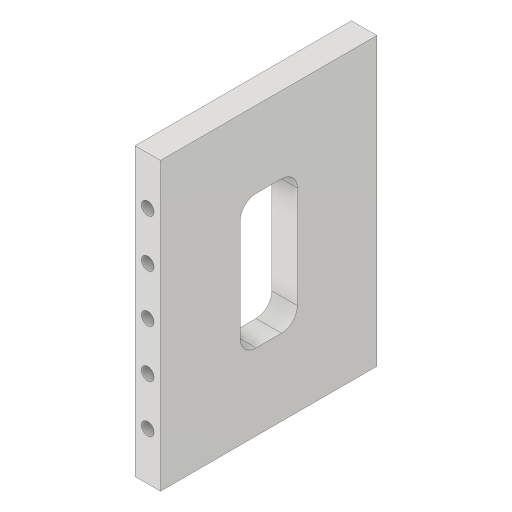
# Autodesk Inventor part: Box_Side
Saved by Autodesk Inventor 2023.2 (Build 272271000, 271)
## iProperties
Created: 2021-07-28
Part Number: Box_Side
Material: LCP 플라스틱
Document SubType Name: Modeling
Designer: user
Density: 1.626 g/cm^3
Appearance: 매끄러움 - 흰색
Mass: 8.3481 g
Surface Area: 40.5022 cm^2
Volume: 5.13413 cm^3
Author: user
Autodesk Inventor part; units mm, degrees
ref_plane "YZ Plane" through (0, 0, 0) normal (1, 0, 0) x (0, 1, 0)
ref_plane "XZ Plane" through (0, 0, 0) normal (0, 1, 0) x (-1, 0, 0)
ref_plane "XY Plane" through (0, 0, 0) normal (0, 0, 1) x (1, 0, 0)
sketch "스케치1" plane through (0, 0, 0) normal (0, 0, 1) x (1, 0, 0)
  line L0 (-2, 22.5) -> (2, 22.5)
  line L1 (2, 22.5) -> (2, -22.5)
  line L2 (2, -22.5) -> (-2, -22.5)
  line L3 (-2, -22.5) -> (-2, 22.5)
  point P0 (0, 0)
  dimension "d0" = 4
  dimension "d1" = 45
  dimension "d2" = 2
  dimension "d3" = 22.5
  constraints: 8 end point, 2 parallel, 1 horizontal, 1 perpendicular
  measures "d0" distance of L1.end L2.end
  measures "d1" distance of L0.end L1.end
  measures "d2" distance from line of L3 point (0, 0)
  measures "d3" distance from line of point (0, 0) L0
extrude "돌출1" add sketch "스케치1" along normal blind 34
sketch "스케치2" plane through (0, 0, 34) normal (0, 0, 1) x (1, 0, 0)
  circle A0 centre (0, 15) radius 1
  circle A1 centre (0, 7.5) radius 1
  circle A2 centre (0, -7.5) radius 1
  circle A3 centre (0, -15) radius 1
  line L0 (2, 22.5) -> (-2, 22.5) projected
  line L1 (-2, 22.5) -> (-2, -22.5) projected
  line L2 (-2, -22.5) -> (2, -22.5) projected
  line L3 (2, -22.5) -> (2, 22.5) projected
  circle A4 centre (0, 0) radius 1
  point P0 (0, 0)
  dimension "d6" = 2
  dimension "d7" = 2
  dimension "d8" = 2
  dimension "d9" = 2
  dimension "d11" = 2
  dimension "d12" = 2
  dimension "d13" = 2
  dimension "d14" = 2
  dimension "d17" = 7.5
  dimension "d18" = 7.5
  dimension "d20" = 7.5
  dimension "d21" = 2
  dimension "d22" = 2
  dimension "d23" = 7.5
  dimension "d26" = 7.5
  dimension "d27" = 7.5
  constraints: 5 centre point
  measures "d6" diameter of A0
  measures "d7" diameter of A1
  measures "d8" diameter of A2
  measures "d9" diameter of A3
  measures "d11" distance from line of L3 A0.centre
  measures "d12" distance from line of L3 A1.centre
  measures "d13" distance from line of L3 A2.centre
  measures "d14" distance from line of L3 A3.centre
  measures "d17" distance from line of A0.centre L0
  measures "d18" distance of A1.centre A0.centre
  measures "d20" distance of A3.centre A2.centre
  measures "d21" distance from line of L3 A4.centre
  measures "d22" diameter of A4
  measures "d23" distance of A1.centre A4.centre
  measures "d26" distance from line of L2 A3.centre
  measures "d27" distance of A2.centre point (0, 0)
extrude "돌출3" cut sketch "스케치2" against normal blind 8 contours A0 | A1 | A2 | A3 | A4
sketch "스케치3" plane through (0, 0, 0) normal (0, 0, -1) x (-1, 0, 0)
  circle A0 centre (0, -15) radius 1 projected
  circle A1 centre (0, 7.5) radius 1 projected
  circle A2 centre (0, 15) radius 1 projected
  circle A3 centre (0, -7.5) radius 1 projected
  circle A4 centre (0, 0) radius 1 projected
  line L0 (-2, 22.5) -> (2, 22.5) projected
  line L1 (2, 22.5) -> (2, -22.5) projected
  line L2 (2, -22.5) -> (-2, -22.5) projected
  line L3 (-2, -22.5) -> (-2, 22.5) projected
  point P0 (0, 0)
extrude "돌출4" cut sketch "스케치3" against normal blind 8 contours A0 | A1 | A2 | A3 | A4
sketch "스케치4" plane through (-2, -22.5, 0) normal (-1, 0, 0) x (0, 0, 1)
  line L0 (0, 0) -> (0, 45) projected
  line L1 (0, 0) -> (34, 0) projected
  line L2 (34, 45) -> (34, 0) projected
  line L3 (0, 45) -> (34, 45) projected
  line L4 (8, 36.5) -> (8, 38.5) projected
  line L5 (26, 38.5) -> (26, 36.5) projected
  line L6 (12.5, 33) -> (21.5, 33)
  line L7 (21.5, 33) -> (21.5, 12)
  line L8 (21.5, 12) -> (12.5, 12)
  line L9 (12.5, 12) -> (12.5, 33)
  point P0 (0, 22.5)
  dimension "d32" = 12
  dimension "d33" = 21
  dimension "d34" = 9
  dimension "d35" = 12.5
  dimension "d36" = 34
  dimension "d37" = 12.5
  dimension "d40" = 45
  dimension "d41" = 12
  constraints: 8 end point, 2 parallel, 1 horizontal, 1 perpendicular
  measures "d32" distance between parallel lines of L6 L3
  measures "d33" distance between parallel lines of L8 L6
  measures "d34" distance between parallel lines of L7 L9
  measures "d35" distance between parallel lines of L0 L9
  measures "d36" distance between parallel lines of L2 L0
  measures "d37" distance between parallel lines of L2 L7
  measures "d40" distance between parallel lines of L1 L3
  measures "d41" distance between parallel lines of L1 L8
extrude "돌출5" cut sketch "스케치4" against normal up to surface (4 mm away) contours L6 L7 L8 L9
fillet "모깎기1" radius 2.5 4 edges at (0, 10.5, 12.5) (0, 10.5, 21.5) (0, -10.5, 12.5) (0, -10.5, 21.5)
equation "\"d2\" = 0.5 * d0"
equation "\"d3\" = 0.5 * d1"
equation "\"d35\" = -0.5 * d34 + 0.5 * d36"
